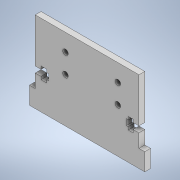
# Autodesk Inventor part: Muñeca1
Saved by Autodesk Inventor 2022 (Build 260153000, 153)
## iProperties
Created: 2021-09-13
Part Number: Muñeca1
Material: Generic
Document SubType Name: Modeling
Designer: Administrador
Density: 1 g/cm^3
Appearance: Default
Author: Administrador
Autodesk Inventor part; units mm, degrees
ref_plane "YZ Plane" through (0, 0, 0) normal (1, 0, 0) x (0, 1, 0)
ref_plane "XZ Plane" through (0, 0, 0) normal (0, 1, 0) x (-1, 0, 0)
ref_plane "XY Plane" through (0, 0, 0) normal (0, 0, 1) x (1, 0, 0)
sketch "Sketch1" plane through (0, 0, 0) normal (0, 0, 1) x (1, 0, 0)
  line L0 (50, 15.95) -> (50, 19.05)
  line L1 (56.5, 15.95) -> (53.5, 15.95)
  line L2 (51, 15.95) -> (51, 15.95)
  line L3 (53.5, 14.45) -> (51, 14.45)
  line L4 (51, 20.55) -> (53.5, 20.55)
  line L5 (51, 14.45) -> (51, 15.95)
  line L6 (51, 19.05) -> (51, 20.55)
  line L7 (50, 19.05) -> (51, 19.05)
  line L8 (53.5, 19.05) -> (56.5, 19.05)
  line L9 (56.5, 15.95) -> (53.5, 15.95)
  line L10 (51, 15.95) -> (50, 15.95)
  line L11 (53.5, 20.55) -> (53.5, 19.05)
  line L12 (53.5, 15.95) -> (53.5, 14.45)
  line L13 (10, 15.95) -> (10, 19.05)
  line L14 (10, 19.05) -> (9, 19.05)
  line L15 (9, 14.45) -> (9, 15.95)
  line L16 (9, 19.05) -> (9, 20.55)
  line L17 (6, 20.55) -> (6, 19.05)
  line L18 (9, 20.55) -> (6, 20.55)
  line L19 (6, 15.95) -> (6, 14.45)
  line L20 (6, 19.05) -> (3, 19.05)
  line L21 (3, 15.95) -> (6, 15.95)
  line L22 (3, 15.95) -> (6, 15.95)
  line L23 (6, 14.45) -> (9, 14.45)
  line L24 (56.5, 19.05) -> (56.5, 41.9)
  line L25 (3, 15.95) -> (3, 9)
  line L26 (3, 9) -> (0, 9)
  line L27 (0, 9) -> (0, 0)
  line L28 (3, 19.05) -> (3, 41.9)
  line L29 (56.5, 41.9) -> (3, 41.9)
  line L30 (9, 15.95) -> (10, 15.95)
  line L31 (56.5, 15.95) -> (56.5, 9)
  line L32 (56.5, 9) -> (59.5, 9)
  line L33 (59.5, 9) -> (59.5, 0)
  line L34 (59.5, 0) -> (0, 0)
  circle A0 centre (45.6295, 23.05) radius 1.425 projected
  circle A1 centre (18.6295, 23.05) radius 1.425 projected
  circle A2 centre (18.6295, 33) radius 1.425 projected
  circle A3 centre (45.6295, 33) radius 1.425 projected
  circle A4 centre (45.6295, 23.05) radius 1.425
  circle A5 centre (45.6295, 33) radius 1.425
  circle A6 centre (18.6295, 33) radius 1.425
  circle A7 centre (18.6295, 23.05) radius 1.425
  line L35 (59.5, 9) -> (59.5, 17.5) construction
  line L36 (59.5, 17.5) -> (59.5, 15.95) construction
  line L37 (59.5, 15.95) -> (56.5, 15.95) construction
  dimension "d54" = 3.1
  dimension "d70" = 3.1
  dimension "d74" = 1.5
  dimension "d83" = 3
  dimension "d85" = 3.1
  dimension "d87" = 3
  dimension "d100" = 9
  dimension "d102" = 3.1
  dimension "d103" = 0
  dimension "d104" = 0
  dimension "d105" = 53.5
  dimension "d108" = 3
  dimension "d109" = 9
  dimension "d110" = 9
  dimension "d111" = 0
  dimension "d112" = 3
  dimension "d113" = 3
  dimension "d114" = 2.5
  dimension "d115" = 1
  dimension "d116" = 1
  dimension "d117" = 1.5
  dimension "d121" = 8.5
  dimension "d122" = 1.55
  dimension "d123" = 6.95
  dimension "d124" = 6.95
  dimension "d125" = 1
  dimension "d126" = 1
  dimension "d127" = 3
  dimension "d128" = 3
  dimension "d129" = 1.5
  dimension "d130" = 1.5
  dimension "d131" = 0
  dimension "d132" = 1.5
  dimension "d133" = 1.5
  dimension "d134" = 1.5
  dimension "d136" = 27
  constraints: 76 end point, 13 perpendicular, 5 coincident, 5 parallel, 4 centre point, 4 concentric, 4 vertical, 3 horizontal, 2 point on line
  measures "d54" distance of L0.start L0.end
  measures "d70" distance between parallel lines of L8 L1
  measures "d74" distance of L4.end L8.start
  measures "d83" distance of L23.start L15.start
  measures "d85" distance of L13.start L13.end
  measures "d87" distance of L16.end L17.start
  measures "d100" distance of L26.end L27.end
  measures "d102" distance between parallel lines of L20 L21
  measures "d103" distance of L27.end point (0, 0)
  measures "d104" distance of point (0, 0) L27.end
  measures "d105" distance of L24.end L28.end
  measures "d108" distance of L31.end L32.end
  measures "d109" distance between parallel lines of L34 L32
  measures "d110" distance between parallel lines of L34 L26
  measures "d111" distance from line of L2.end L1
  measures "d112" distance of L1.start L1.end
  measures "d113" distance of L8.start L8.end
  measures "d114" distance of L3.start L3.end
  measures "d115" distance between parallel lines of L5 L0
  measures "d116" distance between parallel lines of L0 L6
  measures "d117" distance of L1.end L3.start
  measures "d121" distance of L32.end L35.end
  measures "d122" distance of L35.end L36.end
  measures "d123" distance of L31.end L1.start
  measures "d124" distance of L21.start L25.end
  measures "d125" distance between parallel lines of L13 L15
  measures "d126" distance between parallel lines of L13 L16
  measures "d127" distance between parallel lines of L28 L17
  measures "d128" distance between parallel lines of L25 L19
  measures "d129" distance of L23.start L19.start
  measures "d130" distance between parallel lines of L14 L18
  measures "d131" distance between parallel lines of L22 L30
  measures "d132" distance of L15.start L15.end
  measures "d133" distance of L14.end L16.end
  measures "d134" distance of L17.start L17.end
  measures "d136" distance of A2.centre A3.centre
extrude "Extrusion1" add sketch "Sketch1" along normal blind 3
body "Solid1"
